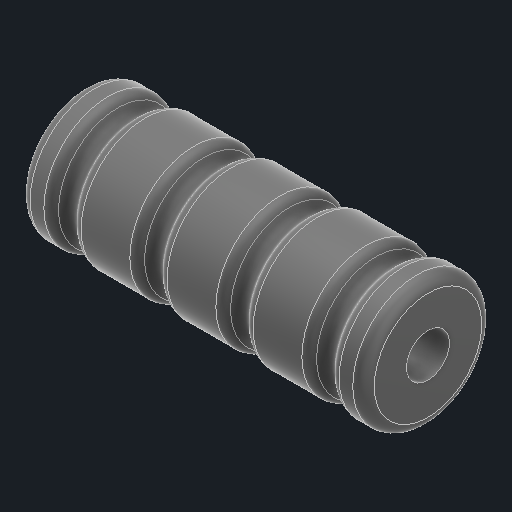
# Autodesk Inventor part: Landing_Foam
Saved by Autodesk Inventor 2025 (Build 290162010, 162A)
## iProperties
Created: 2023-12-05
Part Number: Landing_Foam
Material: Polystyrene, High Impact
Document SubType Name: Modeling
Designer: dzw04
Mass: 47.6076 g
Surface Area: 118.637 cm^2
Volume: 46.5828 cm^3
Density: 1.022 g/cm^3
Appearance: Smooth - Black
Author: dzw04
Autodesk Inventor part; units mm, degrees
ref_plane "YZ Plane" through (0, 0, 0) normal (1, 0, 0) x (0, 1, 0)
ref_plane "XZ Plane" through (0, 0, 0) normal (0, 1, 0) x (-1, 0, 0)
ref_plane "XY Plane" through (0, 0, 0) normal (0, 0, 1) x (1, 0, 0)
sketch "Sketch1" plane through (0, 0, 0) normal (0, 1, 0) x (-1, 0, 0)
  line L0 (40, 0) -> (-40, 0)
  line L1 (40, 5) -> (-40, 5)
  line L2 (-40, 5) -> (-40, 12.5)
  line L3 (-37.5, 15) -> (37.5, 15)
  line L4 (40, 12.5) -> (40, 5)
  circle A0 centre (-30, 15) radius 2.5
  circle A1 centre (-10, 15) radius 2.5
  circle A2 centre (10, 15) radius 2.5
  circle A3 centre (30, 15) radius 2.5
  arc A4 (-37.5, 15) -> (-40, 12.5) centre (-37.5, 12.5) ccw
  arc A5 (40, 12.5) -> (37.5, 15) centre (37.5, 12.5) ccw
  point P0 (0, 0)
  point P1 (0, 0)
  point P2 (-40, 15)
  point P3 (40, 15)
  point P4 (32.5, 15)
  point P5 (27.5, 15)
  point P6 (12.5, 15)
  point P7 (7.5, 15)
  point P8 (-7.5, 15)
  point P9 (-12.5, 15)
  point P10 (-27.5, 15)
  point P11 (-32.5, 15)
  dimension "d0" = 80
  dimension "d1" = 80
  dimension "d2" = 10
  dimension "d4" = 5
  dimension "d5" = 5
  dimension "d6" = 5
  dimension "d7" = 5
  dimension "D1" = 20
  dimension "d9" = 20
  dimension "d10" = 20
  dimension "d11" = 10
  dimension "d12" = 2.5
  dimension "d14" = 10
  constraints: 10 end point, 9 point on line, 6 centre point, 4 point on circle, 4 tangent, 2 horizontal, 2 parallel, 1 coincident, 1 equal radius, 1 midpoint, 1 perpendicular
  measures "d0" distance of L0.start L0.end
  measures "d1" distance of point (-40, 15) point (40, 15)
  measures "d2" distance of L1.end point (-40, 15)
  measures "d4" diameter of A0
  measures "d5" diameter of A1
  measures "d6" diameter of A2
  measures "d7" diameter of A3
  measures "D1" distance of A1.centre A0.centre
  measures "d9" distance of A2.centre A1.centre
  measures "d10" distance of A3.centre A2.centre
  measures "d11" distance of point (-40, 15) A0.centre
  measures "d12" radius of A4
  measures "d14" diameter of L1 L0
revolve "Revolution1" add sketch "Sketch1" angle 360 about axis through (-40, 0, 0) along (1, 0, 0) contours L1 L2 A4 L3 A0 A1 A2 A3 A5 L4
fillet "Fillet1" radius 2.5 8 edges at (32.5, 0, -15) (27.5, 0, -15) (12.5, 0, -15) (7.5, 0, -15) (-7.5, 0, -15) (-12.5, 0, -15) (-27.5, 0, -15) (-32.5, 0, -15)
equation "\"d9\" = D1"
equation "\"d10\" = D1"
equation "\"d11\" = 0.5 * D1"
body "Solid1"
